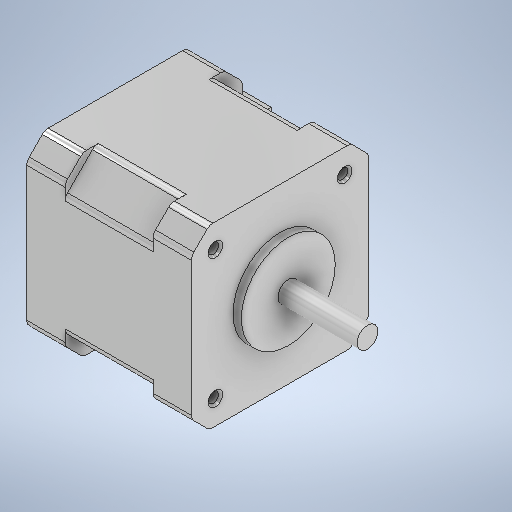
# Autodesk Inventor part: stepper_motor
Saved by Autodesk Inventor 2025 (Build 290162000, 162)
## iProperties
Created: 2024-01-10
Part Number: stepper_motor
Material: 一般
Document SubType Name: Modeling
Designer: 8326d
Density: 1 g/cm^3
Appearance: アルミニウム - ダーク
Author: 8326d
Autodesk Inventor part; units mm, degrees
ref_plane "YZ Plane" through (0, 0, 0) normal (1, 0, 0) x (0, 1, 0)
ref_plane "XZ Plane" through (0, 0, 0) normal (0, 1, 0) x (-1, 0, 0)
ref_plane "XY Plane" through (0, 0, 0) normal (0, 0, 1) x (1, 0, 0)
sketch "スケッチ1" plane through (0, 0, 0) normal (1, 0, 0) x (0, 1, 0)
  line L0 (-21.25, 21.25) -> (21.25, 21.25)
  line L1 (21.25, 21.25) -> (21.25, -21.25)
  line L2 (21.25, -21.25) -> (-21.25, -21.25)
  line L3 (-21.25, -21.25) -> (-21.25, 21.25)
  line L4 (-21.25, 21.25) -> (21.25, -21.25) construction
  line L5 (21.25, 21.25) -> (-21.25, -21.25) construction
  line L6 (16.9338, 21.25) -> (21.25, 16.9338)
  line L7 (21.25, -16.9338) -> (16.9338, -21.25)
  line L8 (-16.9338, -21.25) -> (-21.25, -16.9338)
  line L9 (-21.25, 16.9338) -> (-15.808, 22.3758)
  point P0 (0, 0)
  point P1 (0, 0)
  point P2 (0, 0)
  point P3 (-16.9338, 21.25)
  dimension "d0" = 42.5
  dimension "d1" = 42.5
  dimension "d2" = 27
  dimension "d3" = 27
  dimension "d4" = 27
  dimension "d5" = 27
  constraints: 20 end point, 7 point on line, 4 midpoint, 4 perpendicular, 3 parallel, 1 horizontal
  measures "d0" distance of L1.end L2.end
  measures "d1" distance of L0.end L1.end
  measures "d2" distance from line of L6 point (0, 0)
  measures "d3" distance from line of L8 point (0, 0)
  measures "d4" distance from line of point (0, 0) L7
  measures "d5" distance from line of L9 point (0, 0)
extrude "押し出し1" add sketch "スケッチ1" along normal blind 9.2 contours L6 L1 L7 L2 L8 L3 L9 L0
sketch "スケッチ2" plane through (9.2, 0, 0) normal (1, 0, 0) x (0, 0, -1)
  line L0 (16.9338, 21.25) -> (-16.9338, 21.25) projected
  line L1 (-21.25, 16.9338) -> (-21.25, -16.9338) projected
  line L2 (-16.9338, -21.25) -> (16.9338, -21.25) projected
  line L3 (21.25, -16.9338) -> (21.25, 16.9338) projected
  line L4 (-21.25, 14.1053) -> (-14.1053, 21.25)
  line L5 (14.1053, 21.25) -> (21.25, 14.1053)
  line L6 (21.25, -14.1053) -> (14.1053, -21.25)
  line L7 (-14.1053, -21.25) -> (-21.25, -14.1053)
  point P0 (0, 0)
  dimension "d8" = 25
  dimension "d9" = 25
  dimension "d10" = 25
  dimension "d11" = 25
  dimension "d12" = 135
  constraints: 8 end point, 8 point on line, 3 perpendicular
  measures "d8" distance from line of L4 point (0, 0)
  measures "d9" distance from line of L5 point (0, 0)
  measures "d10" distance from line of point (0, 0) L6
  measures "d11" distance from line of L7 point (0, 0)
  measures "d12" angle of L4 L0
extrude "押し出し2" add sketch "スケッチ2" along normal blind 21.1
sketch "スケッチ3" plane through (30.3, 0, 0) normal (1, 0, 0) x (0, 0, -1)
  line L0 (-16.9338, -21.25) -> (16.9338, -21.25) projected
  line L1 (-21.25, -16.9338) -> (-16.9338, -21.25) projected
  line L2 (-21.25, 16.9338) -> (-21.25, -16.9338) projected
  line L3 (-16.9338, 21.25) -> (-21.25, 16.9338) projected
  line L4 (16.9338, 21.25) -> (-16.9338, 21.25) projected
  line L5 (21.25, 16.9338) -> (16.9338, 21.25) projected
  line L6 (21.25, -16.9338) -> (21.25, 16.9338) projected
  line L7 (16.9338, -21.25) -> (21.25, -16.9338) projected
  point P0 (0, 0)
extrude "押し出し3" add sketch "スケッチ3" along normal blind 9.2
sketch "スケッチ4" plane through (0, 0, 0) normal (-1, 0, 0) x (0, 0, 1)
  line L0 (15.5, 15.5) -> (-15.5, 15.5) construction
  line L1 (-15.5, 15.5) -> (-15.5, -15.5) construction
  line L2 (-15.5, -15.5) -> (15.5, -15.5) construction
  line L3 (15.5, -15.5) -> (15.5, 15.5) construction
  line L4 (15.5, 15.5) -> (-15.5, -15.5) construction
  line L5 (-15.5, 15.5) -> (15.5, -15.5) construction
  point P0 (0, 0)
  dimension "d17" = 31
  dimension "d18" = 31
  constraints: 12 end point, 2 midpoint, 2 parallel, 1 horizontal, 1 perpendicular
  measures "d17" distance of L2.end L1.end
  measures "d18" distance of L1.end L0.end
hole "穴1" at (0, 15.5, -15.5) at (0, -15.5, -15.5) at (0, -15.5, 15.5) at (0, 15.5, 15.5) direction (1, 0, 0) diameter 2.5 depth 8 tip angle 118
chamfer "面取り1" distance 0.5 angle 45 4 edges at (0, -15.5, -16.75) (0, 15.5, -16.75) (0, -15.5, 14.25) (0, 15.5, 14.25)
thread "ねじ1" size "M3x0.5" class "6H" standard "ISO Metric profile" full length
thread "ねじ3" size "M3x0.5" class "6H" standard "ISO Metric profile" full length
thread "ねじ4" size "M3x0.5" class "6H" standard "ISO Metric profile" full length
thread "ねじ5" size "M3x0.5" class "6H" standard "ISO Metric profile" full length
sketch "スケッチ5" plane through (39.5, 0, 0) normal (1, 0, 0) x (0, 0, -1)
  line L0 (-15.5, -15.5) -> (15.5, -15.5) construction
  line L1 (15.5, -15.5) -> (15.5, 15.5) construction
  line L2 (15.5, 15.5) -> (-15.5, 15.5) construction
  line L3 (-15.5, 15.5) -> (-15.5, -15.5) construction
  line L4 (-15.5, -15.5) -> (15.5, 15.5) construction
  line L5 (15.5, -15.5) -> (-15.5, 15.5) construction
  point P0 (0, 0)
  dimension "d31" = 31
  dimension "d32" = 31
  constraints: 12 end point, 2 midpoint, 2 parallel, 1 horizontal, 1 perpendicular
  measures "d31" distance of L2.end L1.end
  measures "d32" distance of L1.end L0.end
hole "穴2" at (39.5, -15.5, 15.5) at (39.5, -15.5, -15.5) at (39.5, 15.5, -15.5) at (39.5, 15.5, 15.5) direction (-1, 0, 0) diameter 2.5 depth 8 tip angle 118
chamfer "面取り2" distance 0.5 angle 45 4 edges at (39.5, -15.5, 16.75) (39.5, -15.5, -14.25) (39.5, 15.5, 16.75) (39.5, 15.5, -14.25)
thread "ねじ2" size "M3x0.5" class "6H" standard "ISO Metric profile" full length
thread "ねじ6" size "M3x0.5" class "6H" standard "ISO Metric profile" full length
thread "ねじ7" size "M2.6x0.45" class "6H" standard "ISO Metric profile" full length
thread "ねじ8" size "M3x0.5" class "6H" standard "ISO Metric profile" full length
sketch "スケッチ6" plane through (39.5, 0, 0) normal (1, 0, 0) x (0, 0, -1)
  circle A0 centre (0, 0) radius 11.25
  dimension "d57" = 22.5
  constraints: 1 centre point, 1 coincident
  measures "d57" diameter of A0
extrude "押し出し4" add sketch "スケッチ6" along normal blind 2
sketch "スケッチ7" plane through (41.5, 0, 0) normal (1, 0, 0) x (0, 0, -1)
  circle A0 centre (0, 0) radius 2.5
  dimension "d60" = 5
  constraints: 1 centre point, 1 coincident
  measures "d60" diameter of A0
extrude "押し出し5" add sketch "スケッチ7" along normal blind 19
sketch "スケッチ8" plane through (0, 0, 0) normal (-1, 0, 0) x (0, 0, 1)
  circle A0 centre (0, 0) radius 4.5
  dimension "d63" = 9
  constraints: 1 centre point, 1 coincident
  measures "d63" diameter of A0
extrude "押し出し6" cut sketch "スケッチ8" against normal blind 3
sketch "スケッチ14" plane through (0, -16.9338, -21.25) normal (0, 0, -1) x (-1, 0, 0)
  line L0 (0, 0) -> (0, 33.8675) projected
  line L1 (-9.2, 0) -> (-9.2, 2.8284) projected
  line L2 (0, 8.9338) -> (-9.2, 8.9338)
  line L3 (-9.2, 8.9338) -> (-9.2, 24.9338)
  line L4 (-9.2, 24.9338) -> (0, 24.9338)
  line L5 (0, 24.9338) -> (0, 8.9338)
  point P0 (0, 16.9338)
  point P1 (-9.2, 16.9338)
  point P2 (0, 16.9338)
  point P3 (0, 16.9338)
  point P4 (0, 16.9338)
  point P5 (0, 24.9338)
  dimension "d97" = 16
  constraints: 8 end point, 5 midpoint, 2 parallel, 1 coincident, 1 horizontal, 1 perpendicular, 1 point on line, 1 vertical alignment
  measures "d97" distance of L2.end L3.end
extrude "押し出し10" add sketch "スケッチ14" along normal blind 7
fillet "フィレット1" radius 2 24 edges at (34.9, -16.9338, -21.25) (34.9, -21.25, -16.9338) (19.75, -14.1053, -21.25) (19.75, -21.25, -14.1053) (4.6, -16.9338, -21.25) (4.6, -21.25, -16.9338) (19.75, 14.1053, -21.25) (19.75, 21.25, -14.1053) (4.6, 21.25, -16.9338) (4.6, 16.9338, -21.25) (34.9, 16.9338, -21.25) (34.9, 21.25, -16.9338) (4.6, 21.25, 16.9338) (4.6, 16.9338, 21.25) (19.75, 14.1053, 21.25) (19.75, 21.25, 14.1053) (34.9, 21.25, 16.9338) (34.9, 16.9338, 21.25) (19.75, -14.1053, 21.25) (4.6, -16.9338, 21.25) (4.6, -21.25, 16.9338) (19.75, -21.25, 14.1053) (34.9, -16.9338, 21.25) (34.9, -21.25, 16.9338)
equation "\"d3\" = d2"
equation "\"d4\" = d2"
equation "\"d5\" = d2"
equation "\"d9\" = d8"
equation "\"d10\" = d9"
equation "\"d11\" = d8"
